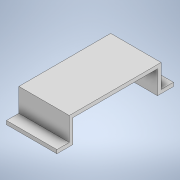
# Autodesk Inventor part: Plastic_Bracket
Saved by Autodesk Inventor 2020 (Build 240168000, 168)
## iProperties
Created: 2019-11-19
Part Number: Plastic_Bracket
Material: Generic
Document SubType Name: Modeling
Designer: kylew
Density: 1 g/cm^3
Appearance: Default
Author: kylew
Autodesk Inventor part; units mm, degrees
ref_plane "YZ Plane" through (0, 0, 0) normal (1, 0, 0) x (0, 1, 0)
ref_plane "XZ Plane" through (0, 0, 0) normal (0, 1, 0) x (-1, 0, 0)
ref_plane "XY Plane" through (0, 0, 0) normal (0, 0, 1) x (1, 0, 0)
sketch "Sketch1" plane through (0, 0, 0) normal (0, 1, 0) x (-1, 0, 0)
  line L0 (34.6, -58) -> (-34.6, -58)
  line L1 (-34.6, -58) -> (-34.6, 58)
  line L2 (-34.6, 58) -> (34.6, 58)
  line L3 (34.6, 58) -> (34.6, -58)
  line L4 (34.6, -58) -> (-34.6, 58) construction
  line L5 (-34.6, -58) -> (34.6, 58) construction
  line L6 (34.6, 80) -> (-34.6, 80)
  line L7 (-34.6, 80) -> (-34.6, -80)
  line L8 (-34.6, -80) -> (34.6, -80)
  line L9 (34.6, -80) -> (34.6, 80)
  line L10 (34.6, 80) -> (-34.6, -80) construction
  line L11 (-34.6, 80) -> (34.6, -80) construction
  line L12 (-34.6, 80) -> (-34.6, -80)
  line L13 (-34.6, -80) -> (-54.6, -80)
  line L14 (-54.6, -80) -> (-54.6, 80)
  line L15 (-54.6, 80) -> (-34.6, 80)
  point P0 (0, 0)
  dimension "d0" = 69.2
  dimension "d1" = 116
  dimension "d2" = 69.2
  dimension "d3" = 160
  dimension "d4" = 20
  constraints: 32 end point, 7 equal length, 4 midpoint, 3 perpendicular, 2 horizontal
  measures "d0" distance of L1.end L2.end
  measures "d1" distance of L0.end L1.end
  measures "d2" distance of L8.end L7.end
  measures "d3" distance of L7.end L6.end
  measures "d4" distance of L7.end L13.end
extrude "Extrusion1" add sketch "Sketch1" along normal blind 5 contours L9 L8 L7 L0 | L2 L7 L6 L9
sketch "Sketch3" plane through (0, 5, 0) normal (0, 1, 0) x (1, 0, 0)
  line L0 (34.6, -58) -> (-34.6, -58) projected
  line L1 (-34.6, -58) -> (34.6, -58)
  line L2 (34.6, -58) -> (34.6, -63)
  line L3 (34.6, -63) -> (-34.6, -63)
  line L4 (-34.6, -63) -> (-34.6, -58)
  line L5 (-34.6, 58) -> (34.6, 58) projected
  line L6 (-34.6, 58) -> (34.6, 58)
  line L7 (34.6, 58) -> (34.6, 63)
  line L8 (34.6, 63) -> (-34.6, 63)
  line L9 (-34.6, 63) -> (-34.6, 58)
  point P0 (0, 0)
  dimension "d7" = 5
  dimension "d8" = 5
  constraints: 16 end point, 4 parallel, 3 perpendicular, 1 horizontal
  measures "d7" distance of L0.start L2.end
  measures "d8" distance of L7.end L5.end
extrude "Extrusion2" add sketch "Sketch3" along normal blind 32
sketch "Sketch4" plane through (0, 37, 0) normal (0, 1, 0) x (1, 0, 0)
  line L0 (34.6, -58) -> (-34.6, -58) projected
  line L1 (-34.6, 58) -> (34.6, 58) projected
  line L2 (-34.6, -58) -> (34.6, -58)
  line L3 (34.6, -58) -> (34.6, 58)
  line L4 (34.6, 58) -> (-34.6, 58)
  line L5 (-34.6, 58) -> (-34.6, -58)
  point P0 (0, 0)
  constraints: 8 end point, 2 parallel, 1 horizontal, 1 perpendicular
extrude "Extrusion3" add sketch "Sketch4" against normal blind 5
body "Solid1"
